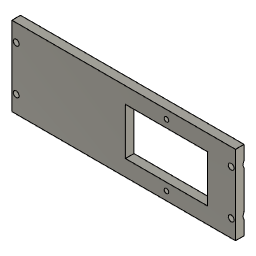
Back Panel v3 (Autodesk Fusion 360 design; units mm, degrees)
Autodesk Fusion 360 part; units mm, degrees
sketch "Sketch1" plane through (0, 0, 0) normal (0, 0, 1) x (1, 0, 0)
  line L0 (0, 0) -> (130, 0)
  line L1 (130, 0) -> (130, 5)
  line L2 (130, 5) -> (0, 5)
  line L3 (0, 5) -> (0, 0)
  dimension "d1" = 130
  dimension "d2" = 5
  constraint horizontal L0
  constraint vertical L1
  constraint horizontal L2
  constraint vertical L3
  constraint coincident L0.start L3.end
  measures "d1" distance of L0.start L0.end
  measures "d2" distance of L0.start L2.end
extrude "Extrude1" add sketch "Sketch1" along normal blind 46
sketch "Sketch3" plane through (0, 5, 0) normal (0, 1, 0) x (-1, 0, 0)
  line L0 (-130, 0) -> (0, 0)
  line L1 (0, 0) -> (0, 46)
  line L2 (0, 46) -> (-130, 46)
  line L3 (-130, 46) -> (-130, 0)
  line L4 (-125, 46) -> (-125, 0) construction
  line L5 (-5, 46) -> (-5, 0) construction
  point P0 (-127.5, 36)
  point P1 (-127.5, 10)
  point P2 (-2.5, 10)
  point P3 (-2.5, 36)
  dimension "d26" = 5
  dimension "d27" = 5
  dimension "d28" = 2.5
  dimension "d29" = 2.5
  dimension "d30" = 10
  dimension "d31" = 10
  dimension "d32" = 10
  dimension "d33" = 10
  dimension "d34" = 2.5
  dimension "d35" = 2.5
  constraint coincident L2 L4.start
  constraint coincident L0 L4.end
  constraint perpendicular L0 L4
  constraint coincident L2 L5.start
  constraint coincident L0 L5.end
  constraint perpendicular L0 L5
  measures "d26" distance of L1 L5
  measures "d27" distance of L3 L4
  measures "d28" distance of L1 P3
  measures "d29" distance of L1 P2
  measures "d30" distance of L0 P2
  measures "d31" distance of L2 P3
  measures "d32" distance of L2 P0
  measures "d33" distance of L0 P1
  measures "d34" distance of L3 P1
  measures "d35" distance of L3 P0
hole "Hole2" at (127.5, 5, 36) at (127.5, 5, 10) at (2.5, 5, 10) at (2.5, 5, 36) direction (0, -1, 0) diameter 3.4 depth 50 tip angle 180 countersink diameter 6.3 countersink angle 90
sketch "Sketch4" plane through (0, 5, 0) normal (0, 1, 0) x (-1, 0, 0)
  arc A0 (0, 11.9164) -> (0, 8.0836) centre (-2.5, 10) ccw
  line L0 (0, 11.9164) -> (0, 34.0836)
  arc A1 (0, 37.9164) -> (0, 34.0836) centre (-2.5, 36) ccw
  line L1 (0, 37.9164) -> (0, 46)
  line L2 (0, 46) -> (-130, 46)
  line L3 (-130, 46) -> (-130, 37.9164)
  arc A2 (-130, 34.0836) -> (-130, 37.9164) centre (-127.5, 36) ccw
  line L4 (-130, 34.0836) -> (-130, 11.9164)
  arc A3 (-130, 8.0836) -> (-130, 11.9164) centre (-127.5, 10) ccw
  line L5 (-130, 8.0836) -> (-130, 0)
  line L6 (-130, 0) -> (0, 0)
  line L7 (0, 0) -> (0, 8.0836)
  line L8 (-113.75, 36.65) -> (-65.95, 36.65)
  line L9 (-65.95, 36.65) -> (-65.95, 9.35)
  line L10 (-65.95, 9.35) -> (-113.75, 9.35)
  line L11 (-113.75, 9.35) -> (-113.75, 36.65)
  line L12 (-130, 23) -> (0, 23) construction
  line L13 (-89.85, 36.65) -> (-89.85, 9.35) construction
  point P0 (-113.75, 23)
  point P1 (-89.85, 41.034)
  point P2 (-89.85, 4.966)
  dimension "d41" = 47.8
  dimension "d42" = 27.3
  dimension "d43" = 18.034
  dimension "d44" = 18.034
  dimension "d51" = 16.25
  constraint horizontal L8
  constraint vertical L9
  constraint horizontal L10
  constraint vertical L11
  constraint midpoint L4 L12.start
  constraint midpoint L0 L12.end
  constraint midpoint L11 P0
  constraint coincident L12 P0
  constraint midpoint L8 L13.start
  constraint midpoint L10 L13.end
  constraint coincident L13 P1
  constraint coincident L13 P2
  measures "d41" distance of L8.start L8.end
  measures "d42" distance of L8.start L10.end
  measures "d43" distance of L12 P1
  measures "d44" distance of L12 P2
  measures "d51" distance of L4 L11
extrude "Extrude2" cut sketch "Sketch4" against normal up to surface (5 mm away) contours L8 L9 L10 L11
hole "Hole3" at (89.85, 5, 41.034) at (89.85, 5, 4.966) direction (0, -1, 0) diameter 2.65 depth 50 tip angle 180
equation "d51 = ( 130 / 8 ) * 1 mm"
